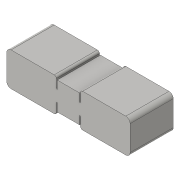
# Autodesk Inventor part: ConnectorNT
Saved by Autodesk Inventor 2016 (Build 200138000, 138)
## iProperties
Created: 2016-01-27
Part Number: ConnectorNT
Material: Generic
Document SubType Name: Modeling
Designer: 301278
Density: 1 g/cm^3
Appearance: Default
Author: 301278
Autodesk Inventor part; units mm, degrees
ref_plane "YZ Plane" through (0, 0, 0) normal (1, 0, 0) x (0, 1, 0)
ref_plane "XZ Plane" through (0, 0, 0) normal (0, 1, 0) x (-1, 0, 0)
ref_plane "XY Plane" through (0, 0, 0) normal (0, 0, 1) x (1, 0, 0)
sketch "Sketch1" plane through (0, 0, 0) normal (0, 0, 1) x (1, 0, 0)
  line L0 (0, 0) -> (0, 8.128)
  line L1 (0, 8.128) -> (-6.604, 8.128)
  line L2 (-6.604, 8.128) -> (-6.604, 3.81)
  arc A0 (-7.112, 3.81) -> (-6.604, 3.302) centre (-6.604, 3.81) ccw
  line L3 (-6.604, 3.81) -> (-6.604, 3.302)
  line L4 (-7.112, 3.81) -> (-7.112, 8.636)
  line L5 (-8.382, 9.906) -> (-33.782, 9.906)
  arc A1 (-7.112, 8.636) -> (-8.382, 9.906) centre (-8.382, 8.636) ccw
  line L6 (-36.322, 7.366) -> (-36.322, 0)
  arc A2 (-33.782, 9.906) -> (-36.322, 7.366) centre (-33.782, 7.366) ccw
  line L7 (0, 8.128) -> (6.604, 8.128)
  line L8 (6.604, 8.128) -> (6.604, 3.81)
  line L9 (7.112, 3.81) -> (7.112, 8.636)
  line L10 (8.382, 9.906) -> (33.782, 9.906)
  arc A3 (8.382, 9.906) -> (7.112, 8.636) centre (8.382, 8.636) ccw
  line L11 (36.322, 7.366) -> (36.322, 0)
  arc A4 (36.322, 7.366) -> (33.782, 9.906) centre (33.782, 7.366) ccw
  line L12 (6.604, 3.81) -> (6.604, 3.302)
  arc A5 (6.604, 3.302) -> (7.112, 3.81) centre (6.604, 3.81) ccw
  line L13 (0, 0) -> (0, -8.128)
  line L14 (0, -8.128) -> (-6.604, -8.128)
  line L15 (-6.604, -8.128) -> (-6.604, -3.81)
  arc A6 (-6.604, -3.302) -> (-7.112, -3.81) centre (-6.604, -3.81) ccw
  line L16 (-6.604, -3.81) -> (-6.604, -3.302)
  line L17 (-7.112, -3.81) -> (-7.112, -8.636)
  line L18 (-8.382, -9.906) -> (-33.782, -9.906)
  arc A7 (-8.382, -9.906) -> (-7.112, -8.636) centre (-8.382, -8.636) ccw
  line L19 (-36.322, -7.366) -> (-36.322, 0)
  arc A8 (-36.322, -7.366) -> (-33.782, -9.906) centre (-33.782, -7.366) ccw
  line L20 (0, -8.128) -> (6.604, -8.128)
  line L21 (6.604, -8.128) -> (6.604, -3.81)
  line L22 (7.112, -3.81) -> (7.112, -8.636)
  arc A9 (7.112, -8.636) -> (8.382, -9.906) centre (8.382, -8.636) ccw
  line L23 (8.382, -9.906) -> (33.782, -9.906)
  arc A10 (33.782, -9.906) -> (36.322, -7.366) centre (33.782, -7.366) ccw
  line L24 (36.322, -7.366) -> (36.322, 0)
  line L25 (6.604, -3.81) -> (6.604, -3.302)
  arc A11 (7.112, -3.81) -> (6.604, -3.302) centre (6.604, -3.81) ccw
  point P0 (-7.112, 9.906)
  point P1 (-36.322, 9.906)
  point P2 (-7.112, -9.906)
  point P3 (-36.322, -9.906)
  dimension "d1" = 6.604
  dimension "d2" = 4.318
  dimension "d3" = 1.016
  dimension "d4" = 6.096
  dimension "d5" = 29.21
  dimension "d6" = 1.27
  dimension "d7" = 9.906
  dimension "d8" = 2.54
  dimension "d9" = 8.128
  constraints: 52 end point, 24 point on circle, 12 centre point, 11 symmetric about line, 8 point on line, 5 tangent, 5 vertical, 2 coincident, 2 perpendicular, 1 horizontal, 3 other
  measures "d1" distance of L0.end L1.end
  measures "d2" distance of L1.end L2.end
  measures "d3" diameter of A0
  measures "d4" distance of L4.start point (-7.112, 9.906)
  measures "d5" distance of point (-7.112, 9.906) point (-36.322, 9.906)
  measures "d6" radius of A1
  measures "d7" distance of point (-36.322, 9.906) L6.end
  measures "d8" radius of A2
  measures "d9" distance of L0.start L0.end
extrude "Extrusion1" add sketch "Sketch1" along normal blind 25.4 contours L0 L7 L8 L12 A5 L9 A3 L10 A4 L11 L24 A10 L23 A9 L22 A11 L25 L21 L20 L13
mirror "Mirror1" about plane through (0, 8.128, 0) normal (-1, 0, 0) of "Extrusion1"
body "Solid1"
